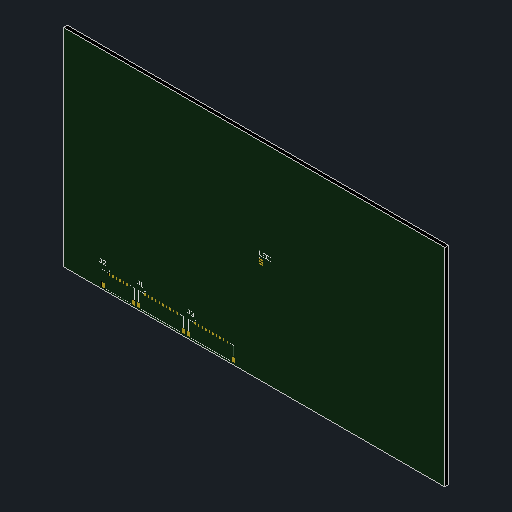
# Autodesk Inventor part: ledbrick_plus_led_BOARD
Saved by Autodesk Inventor 2026.1 (Build 301233020, 233B)
## iProperties
Created: 2025-09-21
Part Number: ledbrick_plus_led_BOARD
Material: Generic
Document SubType Name: Modeling
Designer: atrus
Density: 1 g/cm^3
Appearance: BoardColor
Author: atrus
Autodesk Inventor part; units mm, degrees
ref_plane "YZ Plane" through (0, 0, 0) normal (1, 0, 0) x (0, 1, 0)
ref_plane "XZ Plane" through (0, 0, 0) normal (0, 1, 0) x (-1, 0, 0)
ref_plane "XY Plane" through (0, 0, 0) normal (0, 0, 1) x (1, 0, 0)
ref_plane "BoardFrontPlane" through (0, 0, 0) normal (0, 0, 1) x (1, 0, 0)
sketch "Sketch1" plane through (0, 0, 0) normal (0, 0, 1) x (1, 0, 0)
  line L0 (26, 26) -> (186, 26)
  line L1 (186, 26) -> (186, 113)
  line L2 (186, 113) -> (26, 113)
  line L3 (26, 113) -> (26, 26)
  constraints: 8 end point
extrude "BoardOutline" add sketch "Sketch1" along normal blind 1.5957
sketch "img_Top" plane through (0, 0, 1.5957) normal (0, 0, 1) x (1, 0, 0)
  line L0 (26, 113) -> (186, 113) construction
  line L1 (186, 113) -> (186, 26.0021) construction
  line L2 (186, 26.0021) -> (26, 26.0021) construction
  line L3 (26, 26.0021) -> (26, 113) construction
  constraints: 2 other
decal "Decal_Top"
body "Solid1"
